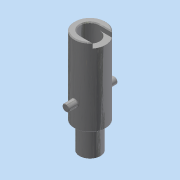
# Autodesk Inventor part: canon
Saved by Autodesk Inventor 2017 (Build 210142000, 142)
## iProperties
Created: 2018-04-15
Part Number: canon
Material: S235JR (E24-2)
Document SubType Name: Modeling
Designer: RozierB
Density: 7.85 g/cm^3
Appearance: Acier
Author: RozierB
Autodesk Inventor part; units mm, degrees
ref_plane "YZ Plane" through (0, 0, 0) normal (1, 0, 0) x (0, 1, 0)
ref_plane "XY Plane" through (0, 0, 0) normal (0, 0, 1) x (1, 0, 0)
sketch "Esquisse3" plane through (0, 0, 0) normal (1, 0, 0) x (0, 1, 0)
  line L0 (17, 0) -> (18, -1)
  line L1 (18, -1) -> (18, -89)
  line L2 (18, -89) -> (17, -90)
  line L3 (17, -90) -> (13, -90)
  line L4 (13, -90) -> (12, -91)
  line L5 (12, -91) -> (12, -120)
  line L6 (12, -120) -> (10, -120)
  line L7 (10, -120) -> (10, -50.25)
  line L8 (11, -50) -> (11, -1)
  line L9 (11, -1) -> (12, 0)
  line L10 (12, 0) -> (17, 0)
  line L11 (0, -144) -> (0, 24) projected
  line L12 (11, -50) -> (10.25, -50)
  line L13 (10.25, -50) -> (10, -50.25)
  point P0 (0, 0)
  dimension "d4" = 1
  dimension "d5" = 1
  dimension "d6" = 11
  dimension "d7" = 10
  dimension "d8" = 1
  dimension "d9" = 1
  dimension "d10" = 18
  dimension "d11" = 50
  dimension "d12" = 40
  dimension "d13" = 1
  dimension "d14" = 1
  dimension "d16" = 1
  dimension "d17" = 1
  dimension "d18" = 30
  dimension "d20" = 0.25
  dimension "d21" = 0.25
  constraints: 26 end point, 5 perpendicular, 1 horizontal, 1 horizontal alignment, 1 parallel, 1 point on line, 1 vertical
  measures "d4" horizontal distance of L0.start L0.end
  measures "d5" horizontal distance of L0.start L0.end
  measures "d6" distance between parallel lines of L11 L8
  measures "d7" distance between parallel lines of L11 L7
  measures "d8" horizontal distance of L8.end L9.end
  measures "d9" horizontal distance of L8.end L9.end
  measures "d10" distance between parallel lines of L11 L1
  measures "d11" distance from line of L10 L8.start
  measures "d12" distance from line of L3 L8.start
  measures "d13" horizontal distance of L1.end L2.end
  measures "d14" horizontal distance of L1.end L2.end
  measures "d16" horizontal distance of L3.end L4.end
  measures "d17" horizontal distance of L3.end L4.end
  measures "d18" distance between parallel lines of L3 L6
  measures "d20" horizontal distance of L12.end L7.end
  measures "d21" horizontal distance of L12.end L7.end
revolve "Révolution1" add sketch "Esquisse3" angle 360 about axis through (0, 0, -10) along (0, 0, 1)
sketch "Esquisse4" plane through (0, 0, 0) normal (1, 0, 0) x (0, 1, 0)
  line L0 (18, -1) -> (18, -89) projected
  line L1 (18, -89) -> (17, -90) projected
  line L2 (17, -90) -> (13, -90) projected
  line L3 (13, -90) -> (12, -91) projected
  line L4 (12, -91) -> (12, -120) projected
  line L5 (12, -120) -> (10, -120) projected
  line L6 (10, -120) -> (10, -50.25) projected
  line L7 (10, -50.25) -> (10.25, -50) projected
  line L8 (10.25, -50) -> (11, -50) projected
  line L9 (11, -50) -> (11, -1) projected
  line L10 (11, -1) -> (12, 0) projected
  line L11 (12, 0) -> (17, 0) projected
  line L12 (17, 0) -> (18, -1) projected
  line L13 (-18, -89) -> (-18, -1) projected
  line L14 (-18, -1) -> (-17, 0) projected
  line L15 (-17, 0) -> (-12, 0) projected
  line L16 (-12, 0) -> (-11, -1) projected
  line L17 (-11, -1) -> (-11, -50) projected
  line L18 (-11, -50) -> (-10.25, -50) projected
  line L19 (-10.25, -50) -> (-10, -50.25) projected
  line L20 (-10, -50.25) -> (-10, -120) projected
  line L21 (-10, -120) -> (-12, -120) projected
  line L22 (-12, -120) -> (-12, -91) projected
  line L23 (-12, -91) -> (-13, -90) projected
  line L24 (-13, -90) -> (-17, -90) projected
  line L25 (-17, -90) -> (-18, -89) projected
  line L26 (12, 0) -> (-12, 0)
  line L27 (11, -50) -> (11, -1) projected
  line L28 (11, -6) -> (-11, -6)
  point P0 (0, 0)
  dimension "d22" = 6
  constraints: 4 end point, 2 point on line, 1 collinear, 1 perpendicular
  measures "d22" distance between parallel lines of L28 L26
extrude "Extrusion3" cut sketch "Esquisse4" along normal up to surface contours L10 L9 L28 L17 L16 L26
ref_plane "Plan de construction1" through (0, -18, -45) normal (0, 1, 0) x (-1, 0, 0)
sketch "Esquisse5" plane through (0, -18, -45) normal (0, 1, 0) x (-1, 0, 0)
  circle A0 centre (0, -19) radius 4
  line L0 (0, -99) -> (0, 69) projected
  point P0 (0, 45)
  point P1 (12.0416, 35)
  point P2 (17, 45)
  dimension "d25" = 8
  dimension "d26" = 64
  constraints: 1 centre point, 1 point on line, 1 other
  measures "d25" diameter of A0
extrude "Extrusion4" add sketch "Esquisse5" along normal blind 2 and the other way blind 10
chamfer "Chanfrein1" distance 0.5 angle 45 4 edges at (-3.0446, -17.7406, -61.4057) (4, -17.5499, -63.9963) (-3.0454, -17.7405, -66.5934) (4, -28, -64)
mirror "Symétrie1" about plane through (0, 0, 0) normal (0, 1, 0) of "Extrusion4", "Chanfrein1"
equation "\"d5\" = d4"
equation "\"d8\" = d4"
equation "\"d9\" = d4"
equation "\"d14\" = d13"
equation "\"d16\" = d13"
equation "\"d17\" = d13"
equation "\"d21\" = d20"
